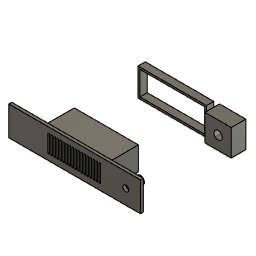
sensor mount (Autodesk Fusion 360 design; units mm, degrees)
Autodesk Fusion 360 part; units mm, degrees
sketch "Sketch1" plane through (0, 0, 0) normal (0, 0, 1) x (1, 0, 0)
  line L0 (0, 0) -> (90, 0)
  line L1 (90, 0) -> (90, 20)
  line L2 (90, 20) -> (0, 20)
  line L3 (0, 20) -> (0, 0)
  line L4 (24.7, 4.1) -> (24.7, 16.1)
  line L5 (64.7, 16.1) -> (64.7, 4.1)
  line L6 (64.7, 4.1) -> (24.7, 16.1) construction
  line L7 (24.7, 4.1) -> (64.7, 16.1) construction
  line L8 (24.7, 16.1) -> (25.7, 16.1)
  line L9 (25.7, 16.1) -> (25.7, 4.1)
  line L10 (25.7, 4.1) -> (24.7, 4.1)
  line L11 (24.7, 4.1) -> (24.7, 16.1)
  line L12 (26.7526, 16.1) -> (27.7526, 16.1)
  line L13 (26.7526, 4.1) -> (26.7526, 16.1)
  line L14 (27.7526, 16.1) -> (27.7526, 4.1)
  line L15 (27.7526, 4.1) -> (26.7526, 4.1)
  line L16 (28.8053, 16.1) -> (29.8053, 16.1)
  line L17 (28.8053, 4.1) -> (28.8053, 16.1)
  line L18 (29.8053, 16.1) -> (29.8053, 4.1)
  line L19 (29.8053, 4.1) -> (28.8053, 4.1)
  line L20 (30.8579, 16.1) -> (31.8579, 16.1)
  line L21 (30.8579, 4.1) -> (30.8579, 16.1)
  line L22 (31.8579, 16.1) -> (31.8579, 4.1)
  line L23 (31.8579, 4.1) -> (30.8579, 4.1)
  line L24 (32.9105, 16.1) -> (33.9105, 16.1)
  line L25 (32.9105, 4.1) -> (32.9105, 16.1)
  line L26 (33.9105, 16.1) -> (33.9105, 4.1)
  line L27 (33.9105, 4.1) -> (32.9105, 4.1)
  line L28 (34.9632, 16.1) -> (35.9632, 16.1)
  line L29 (34.9632, 4.1) -> (34.9632, 16.1)
  line L30 (35.9632, 16.1) -> (35.9632, 4.1)
  line L31 (35.9632, 4.1) -> (34.9632, 4.1)
  line L32 (37.0158, 16.1) -> (38.0158, 16.1)
  line L33 (37.0158, 4.1) -> (37.0158, 16.1)
  line L34 (38.0158, 16.1) -> (38.0158, 4.1)
  line L35 (38.0158, 4.1) -> (37.0158, 4.1)
  line L36 (39.0684, 16.1) -> (40.0684, 16.1)
  line L37 (39.0684, 4.1) -> (39.0684, 16.1)
  line L38 (40.0684, 16.1) -> (40.0684, 4.1)
  line L39 (40.0684, 4.1) -> (39.0684, 4.1)
  line L40 (41.1211, 16.1) -> (42.1211, 16.1)
  line L41 (41.1211, 4.1) -> (41.1211, 16.1)
  line L42 (42.1211, 16.1) -> (42.1211, 4.1)
  line L43 (42.1211, 4.1) -> (41.1211, 4.1)
  line L44 (43.1737, 16.1) -> (44.1737, 16.1)
  line L45 (43.1737, 4.1) -> (43.1737, 16.1)
  line L46 (44.1737, 16.1) -> (44.1737, 4.1)
  line L47 (44.1737, 4.1) -> (43.1737, 4.1)
  line L48 (45.2263, 16.1) -> (46.2263, 16.1)
  line L49 (45.2263, 4.1) -> (45.2263, 16.1)
  line L50 (46.2263, 16.1) -> (46.2263, 4.1)
  line L51 (46.2263, 4.1) -> (45.2263, 4.1)
  line L52 (47.2789, 16.1) -> (48.2789, 16.1)
  line L53 (47.2789, 4.1) -> (47.2789, 16.1)
  line L54 (48.2789, 16.1) -> (48.2789, 4.1)
  line L55 (48.2789, 4.1) -> (47.2789, 4.1)
  line L56 (49.3316, 16.1) -> (50.3316, 16.1)
  line L57 (49.3316, 4.1) -> (49.3316, 16.1)
  line L58 (50.3316, 16.1) -> (50.3316, 4.1)
  line L59 (50.3316, 4.1) -> (49.3316, 4.1)
  line L60 (51.3842, 16.1) -> (52.3842, 16.1)
  line L61 (51.3842, 4.1) -> (51.3842, 16.1)
  line L62 (52.3842, 16.1) -> (52.3842, 4.1)
  line L63 (52.3842, 4.1) -> (51.3842, 4.1)
  line L64 (53.4368, 16.1) -> (54.4368, 16.1)
  line L65 (53.4368, 4.1) -> (53.4368, 16.1)
  line L66 (54.4368, 16.1) -> (54.4368, 4.1)
  line L67 (54.4368, 4.1) -> (53.4368, 4.1)
  line L68 (55.4895, 16.1) -> (56.4895, 16.1)
  line L69 (55.4895, 4.1) -> (55.4895, 16.1)
  line L70 (56.4895, 16.1) -> (56.4895, 4.1)
  line L71 (56.4895, 4.1) -> (55.4895, 4.1)
  line L72 (57.5421, 16.1) -> (58.5421, 16.1)
  line L73 (57.5421, 4.1) -> (57.5421, 16.1)
  line L74 (58.5421, 16.1) -> (58.5421, 4.1)
  line L75 (58.5421, 4.1) -> (57.5421, 4.1)
  line L76 (59.5947, 16.1) -> (60.5947, 16.1)
  line L77 (59.5947, 4.1) -> (59.5947, 16.1)
  line L78 (60.5947, 16.1) -> (60.5947, 4.1)
  line L79 (60.5947, 4.1) -> (59.5947, 4.1)
  line L80 (61.6474, 16.1) -> (62.6474, 16.1)
  line L81 (61.6474, 4.1) -> (61.6474, 16.1)
  line L82 (62.6474, 16.1) -> (62.6474, 4.1)
  line L83 (62.6474, 4.1) -> (61.6474, 4.1)
  line L84 (63.7, 16.1) -> (64.7, 16.1)
  line L85 (63.7, 4.1) -> (63.7, 16.1)
  line L86 (64.7, 16.1) -> (64.7, 4.1)
  line L87 (64.7, 4.1) -> (63.7, 4.1)
  line L88 (63.7, 16.1) -> (64.7, 16.1)
  line L89 (61.6474, 16.1) -> (62.6474, 16.1)
  line L90 (59.5947, 16.1) -> (60.5947, 16.1)
  line L91 (55.4895, 16.1) -> (57.5421, 16.1)
  line L92 (53.4368, 16.1) -> (54.4368, 16.1)
  line L93 (51.3842, 16.1) -> (52.3842, 16.1)
  line L94 (64.7, 4.1) -> (63.7, 4.1)
  line L95 (56.4895, 4.1) -> (55.4895, 4.1)
  line L96 (54.4368, 4.1) -> (53.4368, 4.1)
  line L97 (52.3842, 4.1) -> (51.3842, 4.1)
  line L98 (50.3316, 4.1) -> (49.3316, 4.1)
  line L99 (48.2789, 4.1) -> (47.2789, 4.1)
  line L100 (46.2263, 4.1) -> (45.2263, 4.1)
  line L101 (44.1737, 4.1) -> (43.1737, 4.1)
  line L102 (43.1737, 16.1) -> (44.1737, 16.1)
  line L103 (41.1211, 16.1) -> (42.1211, 16.1)
  line L104 (39.0684, 16.1) -> (40.0684, 16.1)
  line L105 (37.0158, 16.1) -> (38.0158, 16.1)
  line L106 (34.9632, 16.1) -> (35.9632, 16.1)
  line L107 (32.9105, 16.1) -> (33.9105, 16.1)
  line L108 (30.8579, 16.1) -> (31.8579, 16.1)
  line L109 (28.8053, 16.1) -> (29.8053, 16.1)
  line L110 (24.7, 16.1) -> (25.7, 16.1)
  line L111 (26.7526, 16.1) -> (27.7526, 16.1)
  line L112 (25.7, 4.1) -> (24.7, 4.1)
  line L113 (29.8053, 4.1) -> (28.8053, 4.1)
  line L114 (31.8579, 4.1) -> (30.8579, 4.1)
  line L115 (33.9105, 4.1) -> (32.9105, 4.1)
  line L116 (35.9632, 4.1) -> (34.9632, 4.1)
  line L117 (38.0158, 4.1) -> (37.0158, 4.1)
  line L118 (42.1211, 4.1) -> (41.1211, 4.1)
  line L119 (40.0684, 4.1) -> (39.0684, 4.1)
  circle A0 centre (80, 10) radius 2
  line L120 (24.3, 3.65) -> (65.1, 3.65)
  line L121 (65.1, 3.65) -> (65.1, 16.55)
  line L122 (65.1, 16.55) -> (24.3, 16.55)
  line L123 (24.3, 16.55) -> (24.3, 3.65)
  line L124 (24.3, 3.65) -> (65.1, 16.55) construction
  line L125 (65.1, 3.65) -> (24.3, 16.55) construction
  line L126 (22.8, 2.15) -> (66.6, 2.15)
  line L127 (66.6, 2.15) -> (66.6, 18.05)
  line L128 (66.6, 18.05) -> (22.8, 18.05)
  line L129 (22.8, 18.05) -> (22.8, 2.15)
  circle A1 centre (80, 10) radius 2.75
  line L130 (65.1, 16.55) -> (63.9, 16.55)
  line L131 (63.9, 16.55) -> (63.9, 3.65)
  line L132 (63.9, 3.65) -> (65.1, 3.65)
  line L133 (65.1, 3.65) -> (65.1, 16.55)
  line L134 (24.3, 16.55) -> (25.9, 16.55)
  line L135 (25.9, 16.55) -> (25.9, 3.65)
  line L136 (25.9, 3.65) -> (24.3, 3.65)
  line L137 (24.3, 3.65) -> (24.3, 16.55)
  circle A2 centre (80, 10) radius 2.85
  line L138 (71, 1) -> (89, 1)
  line L139 (89, 1) -> (89, 19)
  line L140 (89, 19) -> (71, 19)
  line L141 (71, 19) -> (71, 1)
  line L142 (71, 1) -> (89, 19) construction
  line L143 (89, 1) -> (71, 19) construction
  line L144 (66.8, 18.25) -> (22.6, 18.25)
  line L145 (22.6, 18.25) -> (22.6, 1.95)
  line L146 (22.6, 1.95) -> (66.8, 1.95)
  line L147 (66.8, 1.95) -> (66.8, 18.25)
  line L148 (68.1, 19.55) -> (21.3, 19.55)
  line L149 (21.3, 19.55) -> (21.3, 0.65)
  line L150 (21.3, 0.65) -> (68.1, 0.65)
  line L151 (68.1, 0.65) -> (68.1, 19.55)
  line L152 (68.1, 18.25) -> (68.1, 19.25)
  point P0 (44.7, 10.1)
  point P1 (80, 10)
  dimension "d1" = 90
  dimension "d2" = 20
  dimension "d3" = 40
  dimension "d4" = 12
  dimension "d5" = 1
  dimension "d8" = 39
  dimension "d9" = 40
  dimension "d10" = 4
  dimension "d11" = 10
  dimension "d16" = 40.8
  dimension "d17" = 12.9
  dimension "d18" = 1.5
  dimension "d21" = 5.5
  dimension "d26" = 5.7
  dimension "d27" = 18
  dimension "d28" = 18
  dimension "d65" = 1.7
  dimension "d66" = 3
  dimension "d67" = 1
  constraint horizontal L0
  constraint vertical L1
  constraint horizontal L2
  constraint vertical L3
  constraint coincident L0.start L3.end
  constraint horizontal L94
  constraint perpendicular L4 L94
  constraint parallel L94 L110
  constraint parallel L4 L5
  constraint horizontal L8
  constraint vertical L9
  constraint horizontal L10
  constraint vertical L11
  constraint collinear L88 L110
  constraint collinear L89 L110
  constraint collinear L90 L110
  constraint collinear L91 L110
  constraint collinear L92 L110
  constraint collinear L93 L110
  constraint collinear L95 L96
  constraint collinear L96 L97
  constraint collinear L97 L98
  constraint collinear L98 L99
  constraint collinear L99 L100
  constraint collinear L100 L101
  constraint collinear L101 L118
  constraint collinear L102 L110
  constraint collinear L103 L110
  constraint collinear L104 L110
  constraint collinear L105 L110
  constraint collinear L106 L110
  constraint collinear L107 L110
  constraint collinear L108 L110
  constraint collinear L109 L110
  constraint collinear L110 L111
  constraint collinear L112 L118
  constraint collinear L113 L118
  constraint collinear L114 L118
  constraint collinear L115 L118
  constraint collinear L116 L118
  constraint collinear L117 L118
  constraint collinear L118 L119
  constraint horizontal L120
  constraint perpendicular L120 L121
  constraint parallel L120 L122
  constraint parallel L121 L123
  constraint coincident L124 P0
  constraint coincident L125 P0
  constraint midpoint L6 P0
  constraint concentric A0 A1
  constraint horizontal L130
  constraint vertical L131
  constraint horizontal L132
  constraint vertical L133
  constraint coincident L120 L131.end
  constraint horizontal L134
  constraint vertical L135
  constraint horizontal L136
  constraint vertical L137
  constraint coincident L120 L135.end
  constraint concentric A1 A2
  constraint horizontal L138
  constraint perpendicular L138 L139
  constraint parallel L138 L140
  constraint parallel L139 L141
  constraint coincident L142 P1
  constraint coincident L143 P1
  constraint coincident P1 A0.centre
  constraint coincident L151 L152.start
  constraint perpendicular L144 L152
  measures "d1" distance of L0.start L0.end
  measures "d2" distance of L0.start L2.end
  measures "d3" distance of L4.end L5.start
  measures "d4" distance of L4.start L4.end
  measures "d5" distance of L4.end L8.end
  measures "d10" diameter of A0
  measures "d11" distance of L1 P1
  measures "d16" distance of L121.end L122.end
  measures "d17" distance of L120.end L121.end
  measures "d21" diameter of A1
  measures "d26" diameter of A2
  measures "d27" distance of L139.end L140.end
  measures "d28" distance of L138.end L139.end
  measures "d67" distance of L152.start L152.end
extrude "Extrude1" add sketch "Sketch1" against normal blind 5 contours L148 L149 L150 L151 L152 makes body 1 in component "ramka"
extrude "Extrude1'" add sketch "Sketch1" against normal blind 10 separate body contours L138 L139 L140 L141 makes body 2 in component "temp_sensor"
extrude "Extrude5" add sketch "Sketch1" against normal blind 3 separate body contours L4 L8 L9 L10 L11 L110 L112 | L5 L84 L86 L87 L88 L94 L120 L121 L122 L130 L131 L132 L133 | L5 L84 L86 L87 L88 L94 L131 | L120 L122 L123 L134 L135 L136 L137 makes body 3 at (63.9, 12.25, -1) makes body 4 at (25.9, 12.25, -1)
extrude "Extrude4" add sketch "Sketch1" against normal blind 8 separate body contours A1 makes body 5
extrude "Extrude3" add sketch "Sketch1" against normal blind 20 separate body contours L126 L127 L128 L129 makes body 6
extrude "Extrude2" add sketch "Sketch1" along normal blind 2 separate body contours L0 L1 L2 L3 | L4 L8 L9 L10 L11 L110 L112 | L5 L84 L86 L87 L88 L94 L120 L121 L122 L130 L131 L132 L133 | L5 L84 L86 L87 L88 L94 L131 | L84 L85 L87 L88 L94 L131 | L84 L85 L87 L88 L94 L120 L122 L131 L135 | L120 L122 L123 L134 L135 L136 L137 | L126 L127 L128 L129 | A1 | A2 | L138 L139 L140 L141 | L144 L145 L146 L147 | L148 L149 L150 L151 L152 makes body 7
sketch "Sketch3" plane through (0, 0, -10) normal (0, 0, -1) x (-1, 0, 0)
  circle A0 centre (-80, 10) radius 2.85
  line L0 (-71, 1) -> (-71, 19)
  line L1 (-71, 19) -> (-89, 19)
  line L2 (-89, 19) -> (-89, 1)
  line L3 (-89, 1) -> (-71, 1)
  circle A1 centre (-80, 10) radius 2.5
  circle A2 centre (-74.8, 9) radius 2.25
  circle A3 centre (-74.8, 9) radius 1.2
  circle A4 centre (-85.2, 9) radius 2.25
  circle A5 centre (-85.2, 9) radius 1.2
  line L4 (-85.2, 6) -> (-88.1, 6)
  line L5 (-88.1, 6) -> (-88.1, 17)
  line L6 (-74.8, 6) -> (-71.9, 6)
  line L7 (-85.2, 6) -> (-74.8, 6)
  line L8 (-71.9, 6) -> (-71.9, 17)
  line L9 (-71.9, 17) -> (-88.1, 17)
  line L10 (-85.2, 11.25) -> (-88.1, 11.25)
  line L11 (-82.95, 9) -> (-82.95, 6)
  line L12 (-77.05, 9) -> (-77.05, 6)
  line L13 (-74.8, 11.25) -> (-71.9, 11.25)
  dimension "d33" = 5
  dimension "d36" = 4.5
  dimension "d37" = 2.4
  dimension "d38" = 4.5
  dimension "d39" = 2.4
  dimension "d42" = 2.9
  dimension "d43" = 11
  dimension "d44" = 3
  dimension "d45" = 2.9
  dimension "d46" = 11
  constraint concentric A4 A5
  constraint perpendicular L4 L5
  constraint perpendicular L6 L8
  constraint coincident A4 L10.start
  constraint coincident L5 L10.end
  constraint tangent A4 L10
  constraint perpendicular L5 L10
  constraint coincident A4 L11.start
  constraint coincident L7 L11.end
  constraint tangent A4 L11
  constraint coincident A2 L12.start
  constraint coincident L7 L12.end
  constraint tangent A2 L12
  constraint coincident A2 L13.start
  constraint coincident L8 L13.end
  constraint tangent A2 L13
  constraint perpendicular L8 L13
  measures "d33" diameter of A1
  measures "d36" diameter of A2
  measures "d37" diameter of A3
  measures "d38" diameter of A4
  measures "d39" diameter of A5
  measures "d42" distance of L4.start L4.end
  measures "d43" distance of L4.end L5.end
  measures "d44" distance of A2.centre L6.start
  measures "d45" distance of L6.start L6.end
  measures "d46" distance of L6.end L8.end
extrude "Extrude4'" add sketch "Sketch3" along normal blind 5 contours L0 L1 L2 L3 bodies 2 in component "temp_sensor"
extrude "Extrude3'" add sketch "Sketch3" along normal blind 3 contours A2 | A4 bodies 2 in component "temp_sensor"
extrude "Extrude2'" add sketch "Sketch3" against normal blind 4 contours A0 bodies 2 in component "temp_sensor"
extrude "Extrude5'" add sketch "Sketch3" along normal blind 3 contours A2 L6 L7 L8 L12 L13 | A4 L4 L5 L7 L10 L11 bodies 2 in component "temp_sensor"
extrude "Extrude7" cut 1 faces at (77.3, 17, -11.6667) along direction (0, 1, 0) blind 1 on bodies 2 bodies 2 in component "temp_sensor"
extrude "Extrude9" cut 1 faces at (82.7227, 9.8584, -6) along direction (0, 0, -1) blind 3 on bodies 2 bodies 2 in component "temp_sensor"
extrude "Extrude10" cut 1 faces at (79.929, 3.0527, 0) along direction (0, 0, -1) blind 3 on bodies 2 bodies 2 in component "temp_sensor"
extrude "Extrude11" cut 1 faces at (79.929, 3.0527, -3) along direction (0, 0, -1) blind 2 on bodies 2 bodies 2 in component "temp_sensor"
extrude "Extrude12" cut 1 faces at (82.7227, 9.8584, -9) along direction (0, 0, -1) blind 3.7 on bodies 2 bodies 2 in component "temp_sensor"
ref_plane "WorkPlane1" through (44.7, 68.05, -10) normal (0, 1, 0) x (1, 0, 0)
sketch "Sketch4" plane through (44.7, 68.05, -10) normal (0, 1, 0) x (1, 0, 0)
  line L0 (-13, 3) -> (17, 3)
  line L1 (17, 3) -> (17, -1)
  line L2 (17, -1) -> (-13, -1)
  line L3 (-13, -1) -> (-13, 3)
  dimension "d71" = 30
  dimension "d72" = 4
  constraint horizontal L0
  constraint vertical L1
  constraint horizontal L2
  constraint vertical L3
  measures "d71" distance of L0.start L0.end
  measures "d72" distance of L0.start L2.end
copy_body "CutPasteBodies1" bodies 3 removing the originals makes body 8 in component "grill"
copy_body "CutPasteBodies2" bodies 4 removing the originals makes body 9 in component "grill"
copy_body "CutPasteBodies3" bodies 5 removing the originals makes body 10 in component "grill"
copy_body "CutPasteBodies4" bodies 6 removing the originals makes body 11 in component "grill"
copy_body "CutPasteBodies5" bodies 7 removing the originals makes body 12 in component "grill"
component "temp_sensor" placed x (1, 0, 0) y (0, 1, 0) z (0, 0, 1) at (0, 0, 0)
component "ramka" placed x (1, 0, 0) y (0, 1, 0) z (0, 0, 1) at (0, 0, 0)
component "grill" placed x (1, 0, 0) y (0, 1, 0) z (0, 0, 1) at (0, 0, 0)
